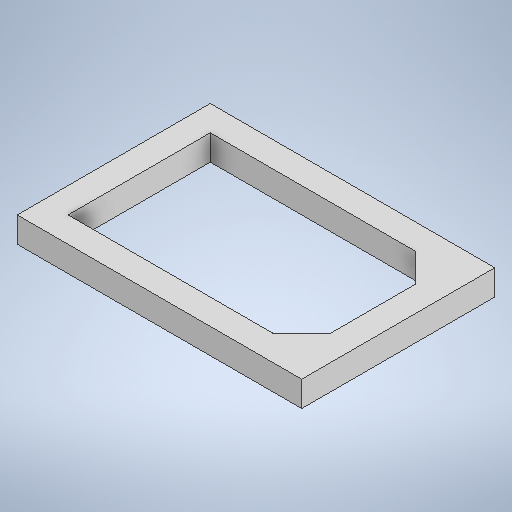
# Autodesk Inventor part: power_test
Saved by Autodesk Inventor 2025 (Build 290162000, 162)
## iProperties
Created: 2024-12-15
Part Number: power_test
Material: Generic
Document SubType Name: Modeling
Designer: ethan
Density: 1 g/cm^3
Appearance: Default
Author: ethan
Autodesk Inventor part; units mm, degrees
ref_plane "YZ Plane" through (0, 0, 0) normal (1, 0, 0) x (0, 1, 0)
ref_plane "XZ Plane" through (0, 0, 0) normal (0, 1, 0) x (-1, 0, 0)
ref_plane "XY Plane" through (0, 0, 0) normal (0, 0, 1) x (1, 0, 0)
sketch "Sketch1" plane through (0, 0, 0) normal (0, 1, 0) x (-1, 0, 0)
  line L0 (5.6569, 0) -> (36, 0)
  line L1 (36, 0) -> (36, -28)
  line L2 (36, -28) -> (5.6569, -28)
  line L3 (0, -28) -> (0, -5.6568)
  line L4 (0, 0) -> (0, -5.6568)
  line L5 (0, -5.6568) -> (5.6569, 0)
  line L6 (36, -14) -> (0, -14) construction
  line L7 (5.6569, -28) -> (36, -28)
  line L8 (0, 0) -> (0, -22.3432)
  line L9 (0, -22.3432) -> (5.6569, -28)
  line L10 (41, -28) -> (41, 5) construction
  line L11 (41, 5) -> (3.5859, 5) construction
  line L12 (3.5859, 5) -> (-3.5355, -2.1212) construction
  line L13 (36, -33) -> (5.6569, -33) construction
  line L14 (36, 0) -> (46, 0) construction
  line L15 (46, 0) -> (46, -28) construction
  line L16 (46, -28) -> (36, -28) construction
  line L17 (36, -28) -> (36, 0) construction
  line L18 (51, 5) -> (31, 5) construction
  line L19 (31, 5) -> (31, -33) construction
  line L20 (31, -33) -> (51, -33) construction
  line L21 (51, -33) -> (51, 5) construction
  line L22 (0, 0) -> (-5, 0) construction
  line L23 (-5, 0) -> (-5, -8.8109) construction
  line L24 (-5, -8.8109) -> (0, -8.8109) construction
  line L25 (0, -8.8109) -> (0, 0) construction
  line L26 (51, 5) -> (-5, 5)
  line L27 (-5, 5) -> (-5, -33.0002)
  line L28 (-5, -33.0002) -> (51, -33.0002)
  line L29 (51, -33.0002) -> (51, 5)
  line L30 (36, 0) -> (46, 0)
  line L31 (46, 0) -> (46, -28)
  line L32 (46, -28) -> (36, -28)
  line L33 (36, -28) -> (36, 0)
  dimension "d0" = 36
  dimension "d1" = 28
  dimension "d3" = 8
  dimension "d4" = 5
  dimension "d5" = 5
  dimension "d6" = 10
  dimension "d7" = 5
  dimension "d8" = 5
  constraints: 68 end point, 13 parallel, 7 perpendicular, 5 horizontal, 2 symmetric about line, 1 midpoint, 1 point on line, 5 other
  measures "d0" distance of L1.end L3.start
  measures "d1" distance of L0.end L1.end
  measures "d3" distance of L0.start L3.end
  measures "d4" distance between parallel lines of L1 L10
  measures "d5" distance between parallel lines of L2 L13
  measures "d6" distance of L15.end L16.end
  measures "d7" distance between parallel lines of L14 L18
  measures "d8" distance of L24.end L23.end
extrude "Extrusion1" add sketch "Sketch1" along normal blind 5
body "Solid1"
